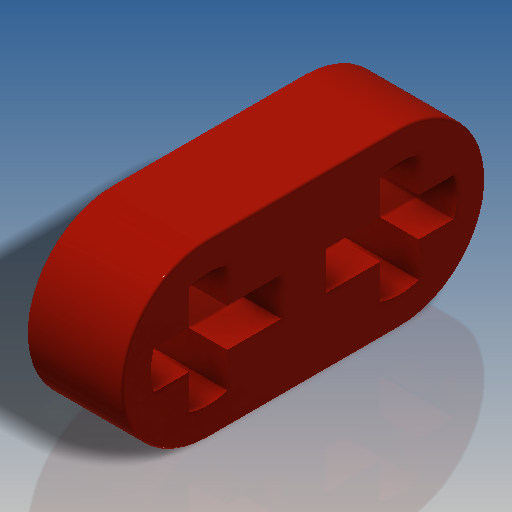
# Autodesk Inventor part: 41677-Red
Saved by Autodesk Inventor 2018.3 (Build 223284000, 284)
## iProperties
Created: 2012-03-28
Part Number: 41677-Red
Document SubType Name: Modeling
Designer: D. Kohfeld
Density: 1.06 g/cm^3
Material: ABS Plastic
Mass: 0.300985 g
Surface Area: 4.51575 cm^2
Volume: 0.283948 cm^3
Appearance: Red
Author: D. Kohfeld
Autodesk Inventor part; units mm, degrees
ref_plane "YZ Plane" through (0, 0, 0) normal (1, 0, 0) x (0, 1, 0)
ref_plane "XZ Plane" through (0, 0, 0) normal (0, 1, 0) x (-1, 0, 0)
ref_plane "XY Plane" through (0, 0, 0) normal (0, 0, 1) x (1, 0, 0)
sketch "Sketch3" plane through (0, 0, 0) normal (1, 0, 0) x (0, 1, 0)
  arc A0 (4.8, 2.2627) -> (3.2, 2.2627) centre (4, 0) ccw
  arc A1 (3.2, -2.2627) -> (4.8, -2.2627) centre (4, 0) ccw
  arc A2 (6.2627, -0.8) -> (6.2627, 0.8) centre (4, 0) ccw
  line L0 (6.2627, 0.8) -> (4.8, 0.8)
  line L1 (3.2, 0.8) -> (1.7373, 0.8)
  line L2 (4.8, 2.2627) -> (4.8, 0.8)
  line L3 (4.8, -0.8) -> (4.8, -2.2627)
  line L4 (6.2627, -0.8) -> (4.8, -0.8)
  line L5 (3.2, -0.8) -> (1.7373, -0.8)
  arc A3 (4, -3.6) -> (4, 3.6) centre (4, 0) ccw
  line L6 (0.9373, -0.8) -> (1.7373, -0.8)
  line L7 (-4, -3.6) -> (4, -3.6)
  line L8 (-4, 3.6) -> (4, 3.6)
  line L9 (3.2, 0.8) -> (3.2, 2.2627)
  line L10 (3.2, -0.8) -> (3.2, -2.2627)
  line L11 (1.7373, 0.8) -> (0.9373, 0.8)
  line L12 (0.9373, 0.8) -> (0.9373, -0.8)
  arc A4 (-4, 3.6) -> (-4, -3.6) centre (-4, 0) ccw
  line L13 (0, -3.6) -> (0, 3.6) construction
  arc A5 (-3.2, 2.2627) -> (-4.8, 2.2627) centre (-4, 0) ccw
  arc A6 (-4.8, -2.2627) -> (-3.2, -2.2627) centre (-4, 0) ccw
  line L14 (-4.8, -0.8) -> (-4.8, -2.2627)
  line L15 (-4.8, 2.2627) -> (-4.8, 0.8)
  line L16 (-6.2627, -0.8) -> (-4.8, -0.8)
  line L17 (-6.2627, 0.8) -> (-4.8, 0.8)
  arc A7 (-6.2627, 0.8) -> (-6.2627, -0.8) centre (-4, 0) ccw
  line L18 (-3.2, 0.8) -> (-1.7373, 0.8)
  line L19 (-0.9373, -0.8) -> (-1.7373, -0.8)
  line L20 (-3.2, -0.8) -> (-1.7373, -0.8)
  line L21 (-3.2, 0.8) -> (-3.2, 2.2627)
  line L22 (-3.2, -0.8) -> (-3.2, -2.2627)
  line L23 (-1.7373, 0.8) -> (-0.9373, 0.8)
  line L24 (-0.9373, 0.8) -> (-0.9373, -0.8)
  point P0 (0, 0)
  dimension "d47" = 4.8
  dimension "d49" = 7.2
  dimension "d53" = 1.6
  dimension "d57" = 0.8
  dimension "d58" = 8
  constraints: 50 end point, 16 point on circle, 16 symmetric about line, 8 centre point, 7 equal length, 7 perpendicular, 6 parallel, 4 tangent, 3 horizontal alignment, 2 coincident, 2 concentric, 2 horizontal, 2 midpoint, 1 collinear, 1 vertical, 1 vertical alignment, 3 other
  measures "d47" diameter of A1
  measures "d49" diameter of A3
  measures "d53" distance between parallel lines of L0 L4
  measures "d57" distance of L6.start L6.end
  measures "d58" distance of A0.centre A4.centre
extrude "Extrusion4" add sketch "Sketch3" along normal mid plane 4
fillet "Fillet1" radius 0.1 6 edges at (-2, 7.6, 0) (-2, 0, 3.6) (-2, 0, -3.6) (2, 0, 3.6) (2, 0, -3.6) (2, 7.6, 0)
equation "\"d47\" = kd"
equation "\"d49\" = tlad"
equation "\"d53\" = axlet"
equation "\"d58\" = lu"
equation "\"d15\" = 0.5 * lu"
equation "\"d56\" = lf"
equation "\"kd\" = 4.8"
equation "\"tlad\" = 7.2"
equation "\"axlet\" = 1.6"
equation "\"lu\" = 8"
equation "\"lf\" = 0.1"
body "Solid1"
